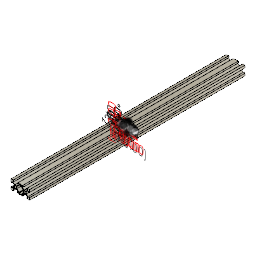
2040-460mm (Autodesk Fusion 360 design; units mm, degrees)
Autodesk Fusion 360 part; units mm, degrees
sketch "Sketch1" plane through (0, 0, 0) normal (0, 1, 0) x (1, 0, 0)
  circle A0 centre (0, 0) radius 2.1
  line L0 (-6.56, 5.4993) -> (-8.2, 5.4993)
  line L1 (-8.2, 5.4993) -> (-8.2, 3.1)
  line L2 (-8.2, 3.1) -> (-10, 4.9)
  line L3 (-10, 4.9) -> (-10, 10)
  line L4 (-10, 10) -> (-4.9, 10)
  line L5 (-4.9, 10) -> (-3.1, 8.2)
  line L6 (-3.1, 8.2) -> (-5.4993, 8.2)
  line L7 (-5.4993, 8.2) -> (-5.4993, 6.56)
  line L8 (-5.4993, 6.56) -> (-1.7793, 2.84)
  line L9 (-6.56, 5.4993) -> (-2.84, 1.7793)
  line L10 (0, 0) -> (-10, 10) construction
  line L11 (0, 0) -> (0, 5) construction
  line L12 (0, 0) -> (-5, 0) construction
  line L13 (-2.84, 1.7793) -> (-2.84, 0)
  line L14 (-1.7793, 2.84) -> (0, 2.84)
  line L15 (-8.2, -3.1) -> (-10, -4.9)
  line L16 (-6.56, -5.4993) -> (-8.2, -5.4993)
  line L17 (-10, -4.9) -> (-10, -10)
  line L18 (-4.9, -10) -> (-3.1, -8.2)
  line L19 (-5.4993, -6.56) -> (-1.7793, -2.84)
  line L20 (-6.56, -5.4993) -> (-2.84, -1.7793)
  line L21 (-1.7793, -2.84) -> (0, -2.84)
  line L22 (-3.1, -8.2) -> (-5.4993, -8.2)
  line L23 (-8.2, -5.4993) -> (-8.2, -3.1)
  line L24 (-10, -10) -> (-4.9, -10)
  line L25 (-5.4993, -8.2) -> (-5.4993, -6.56)
  line L26 (-2.84, -1.7793) -> (-2.84, 0)
  line L27 (4.9, 10) -> (3.1, 8.2)
  line L28 (2.84, -1.7793) -> (2.84, 0)
  line L29 (6.56, -5.4993) -> (2.84, -1.7793)
  line L30 (1.7793, 2.84) -> (0, 2.84)
  line L31 (5.4993, -8.2) -> (5.4993, -6.56)
  line L32 (5.4993, -6.56) -> (1.7793, -2.84)
  line L33 (10, 10) -> (4.9, 10)
  line L34 (2.84, 1.7793) -> (2.84, 0)
  line L35 (3.1, 8.2) -> (5.4993, 8.2)
  line L36 (10, -10) -> (4.9, -10)
  line L37 (1.7793, -2.84) -> (0, -2.84)
  line L38 (5.4993, 6.56) -> (1.7793, 2.84)
  line L39 (4.9, -10) -> (3.1, -8.2)
  line L40 (6.56, 5.4993) -> (2.84, 1.7793)
  line L41 (5.4993, 8.2) -> (5.4993, 6.56)
  line L42 (3.1, -8.2) -> (5.4993, -8.2)
  line L43 (10, -4.9) -> (10, 4.9) construction
  line L44 (20, 0) -> (30, 10) construction
  line L45 (26.56, -5.4993) -> (28.2, -5.4993)
  line L46 (23.1, 8.2) -> (25.4993, 8.2)
  line L47 (30, 4.9) -> (30, 10)
  line L48 (26.56, 5.4993) -> (22.84, 1.7793)
  line L49 (22.84, -1.7793) -> (22.84, 0)
  line L50 (30, -4.9) -> (30, -10)
  line L51 (25.4993, -8.2) -> (25.4993, -6.56)
  line L52 (23.1, -8.2) -> (25.4993, -8.2)
  line L53 (28.2, 5.4993) -> (28.2, 3.1)
  line L54 (28.2, 3.1) -> (30, 4.9)
  line L55 (20, 0) -> (20, 5) construction
  line L56 (20, 0) -> (25, 0) construction
  line L57 (30, -10) -> (24.9, -10)
  line L58 (26.56, -5.4993) -> (22.84, -1.7793)
  line L59 (24.9, -10) -> (23.1, -8.2)
  line L60 (25.4993, 8.2) -> (25.4993, 6.56)
  line L61 (28.2, -3.1) -> (30, -4.9)
  line L62 (22.84, 1.7793) -> (22.84, 0)
  line L63 (28.2, -5.4993) -> (28.2, -3.1)
  line L64 (10, -10) -> (15.1, -10)
  line L65 (16.9, 8.2) -> (14.5007, 8.2)
  line L66 (18.2207, 2.84) -> (20, 2.84)
  line L67 (14.5007, -6.56) -> (18.2207, -2.84)
  line L68 (15.1, 10) -> (16.9, 8.2)
  line L69 (13.44, 5.4993) -> (17.16, 1.7793)
  line L70 (18.2207, -2.84) -> (20, -2.84)
  line L71 (17.16, 1.7793) -> (17.16, 0)
  line L72 (15.1, -10) -> (16.9, -8.2)
  line L73 (14.5007, 6.56) -> (18.2207, 2.84)
  line L74 (17.16, -1.7793) -> (17.16, 0)
  line L75 (21.7793, 2.84) -> (20, 2.84)
  line L76 (30, 10) -> (24.9, 10)
  line L77 (26.56, 5.4993) -> (28.2, 5.4993)
  line L78 (24.9, 10) -> (23.1, 8.2)
  line L79 (25.4993, -6.56) -> (21.7793, -2.84)
  line L80 (14.5007, 8.2) -> (14.5007, 6.56)
  line L81 (10, 10) -> (15.1, 10)
  circle A1 centre (20, 0) radius 2.1
  line L82 (14.5007, -8.2) -> (14.5007, -6.56)
  line L83 (21.7793, -2.84) -> (20, -2.84)
  line L84 (16.9, -8.2) -> (14.5007, -8.2)
  line L85 (25.4993, 6.56) -> (21.7793, 2.84)
  line L86 (13.44, -5.4993) -> (17.16, -1.7793)
  line L87 (6.56, 5.4993) -> (7.2993, 6.2387)
  line L88 (7.2993, 6.2387) -> (7.2993, 8.2)
  line L89 (7.2993, 8.2) -> (12.7007, 8.2)
  line L90 (12.7007, 8.2) -> (12.7007, 6.2387)
  line L91 (12.7007, 6.2387) -> (13.44, 5.4993)
  line L92 (6.56, -5.4993) -> (7.2993, -6.2387)
  line L93 (7.2993, -6.2387) -> (7.2993, -8.2)
  line L94 (7.2993, -8.2) -> (12.7007, -8.2)
  line L95 (12.7007, -8.2) -> (12.7007, -6.2387)
  line L96 (12.7007, -6.2387) -> (13.44, -5.4993)
  point P0 (5, 0)
  point P1 (15, 0)
  point P2 (20, 0)
  point P3 (20, 0)
  dimension "d1" = 4.2
  dimension "d2" = 10
  dimension "d3" = 10
  dimension "d4" = 3.1
  dimension "d5" = 1.8
  dimension "d6" = 0
  dimension "d7" = 1.5
  dimension "d8" = 1.64
  dimension "d9" = 135
  dimension "d10" = 0
  dimension "d11" = 2.84
  dimension "d12" = 0
  dimension "d13" = 0
  dimension "d14" = 20
  dimension "d15" = 0
  dimension "d16" = 0
  constraint coincident A0.centre L10.start
  constraint perpendicular L0 L1
  constraint perpendicular L3 L4
  constraint parallel L2 L5
  constraint perpendicular L3 L6
  constraint perpendicular L6 L7
  constraint vertical L3
  constraint equal L8 L9
  constraint parallel L8 L10
  constraint vertical L11
  constraint perpendicular L11 L12
  constraint coincident L12 L13.end
  constraint perpendicular L12 L13
  constraint coincident L11 L14.end
  constraint perpendicular L11 L14
  constraint symmetric L8.end L9.end L10
  constraint symmetric L0.start L12 L16.start
  constraint symmetric L0.end L12 L16.end
  constraint symmetric L1.end L12 L15.start
  constraint symmetric L2.end L12 L15.end
  constraint symmetric L3.end L12 L17.end
  constraint symmetric L4.end L12 L18.start
  constraint symmetric L5.end L12 L18.end
  constraint symmetric L6.end L12 L22.end
  constraint symmetric L7.end L12 L19.start
  constraint symmetric L8.end L12 L19.end
  constraint symmetric L9.end L12 L20.end
  constraint symmetric L12 L13.end L26.end
  constraint symmetric L12 L14.end L21.end
  constraint symmetric L0.start L11 L40.start
  constraint symmetric L2.end L11 L43.end
  constraint symmetric L3.end L11 L33.start
  constraint symmetric L4.end L11 L27.start
  constraint symmetric L5.end L11 L27.end
  constraint symmetric L6.end L11 L35.end
  constraint symmetric L7.end L11 L38.start
  constraint symmetric L8.end L11 L30.start
  constraint symmetric L9.end L11 L34.start
  constraint symmetric L11 L12.end P0
  constraint symmetric L11 L13.end L28.end
  constraint symmetric L11 L14.end L30.end
  constraint symmetric L11 L17.end L36.start
  constraint symmetric L11 L22.end L31.start
  constraint symmetric L11 L20.end L28.start
  constraint symmetric L11 L15.end L43.start
  constraint symmetric L11 L19.end L32.end
  constraint symmetric L11 L19.start L31.end
  constraint symmetric L11 L18.end L39.end
  constraint symmetric L11 L18.start L36.end
  constraint symmetric L11 L16.start L29.start
  constraint symmetric L11 L21.end L37.end
  constraint symmetric A0.centre L43 P3
  constraint symmetric A0 L43 A1
  constraint symmetric A0.centre L43 P2
  constraint symmetric L0.start L43 L48.start
  constraint symmetric L0.end L43 L53.start
  constraint symmetric L1.end L43 L53.end
  constraint symmetric L2.end L43 L47.start
  constraint symmetric L3.end L43 L44.end
  constraint symmetric L4.end L43 L76.end
  constraint symmetric L5.end L43 L46.start
  constraint symmetric L6.end L43 L46.end
  constraint symmetric L7.end L43 L60.end
  constraint symmetric L8.end L43 L75.start
  constraint symmetric L9.end L43 L48.end
  constraint symmetric L11.end L43 L55.end
  constraint symmetric L12.end L43 L56.end
  constraint symmetric L13.end L43 L49.end
  constraint symmetric L14.end L43 L66.end
  constraint symmetric L16.end L43 L45.end
  constraint symmetric L15.start L43 L61.start
  constraint symmetric L17.end L43 L50.end
  constraint symmetric L22.end L43 L51.start
  constraint symmetric L20.end L43 L49.start
  constraint symmetric L15.end L43 L50.start
  constraint symmetric L19.end L43 L79.end
  constraint symmetric L19.start L43 L51.end
  constraint symmetric L18.end L43 L52.start
  constraint symmetric L18.start L43 L57.end
  constraint symmetric L16.start L43 L45.start
  constraint symmetric L21.end L43 L70.end
  constraint symmetric L31.start L43 L82.start
  constraint symmetric L39.end L43 L72.end
  constraint symmetric L28.end L43 L71.end
  constraint symmetric L29.start L43 L86.start
  constraint symmetric L40.start L43 L69.start
  constraint symmetric L36.end L43 L64.end
  constraint symmetric L31.end L43 L67.start
  constraint symmetric P0 L43 P1
  constraint symmetric L32.end L43 L67.end
  constraint symmetric L28.start L43 L74.start
  constraint symmetric L27.end L43 L65.start
  constraint symmetric L27.start L43 L68.start
  constraint symmetric L36.start L43 L64.start
  constraint symmetric L30.start L43 L66.start
  constraint symmetric L38.start L43 L73.start
  constraint symmetric L35.end L43 L65.end
  constraint symmetric L33.start L43 L81.start
  constraint symmetric L34.start L43 L69.end
  constraint parallel L40 L87
  constraint perpendicular L35 L88
  constraint perpendicular L89 L90
  constraint collinear L69 L91
  constraint collinear L35 L89
  constraint symmetric L12 L40.start L29.start
  constraint symmetric L12 L69.start L86.start
  constraint symmetric L12 L87.end L92.end
  constraint symmetric L12 L88.end L93.end
  constraint symmetric L12 L89.end L94.end
  constraint symmetric L12 L90.end L95.end
  measures "d1" diameter of A0
  measures "d2" distance of A0.centre L4
  measures "d3" distance of A0.centre L3
  measures "d4" vertical distance of A0.centre L1.end
  measures "d5" distance of L1 L3
  measures "d6" distance of L4 L6
  measures "d7" distance of L8 L9
  measures "d8" distance of L6.end L7.end
  measures "d9" angle of L2 L3
  measures "d11" distance of L9.end L11
  measures "d13" distance of L0.start L0.end
  measures "d14" distance of A0.centre P2
  measures "d15" distance of L41 L88
  measures "d16" distance of L80 L90
extrude "Extrude1" add sketch "Sketch1" along normal mid plane 460
equation "d4 = ( 6.2 / 2 ) * 1 mm"
equation "d6 = d10"
equation "d10 = d9"
equation "d11 = ( 5.68 / 2 ) * 1 mm"
equation "d12 = d19"
equation "d13 = d13"
equation "d15 = d10"
equation "d16 = d29"
